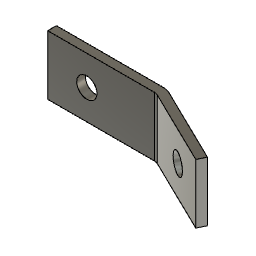
bracket154(2) (Autodesk Fusion 360 design; units mm, degrees)
Autodesk Fusion 360 part; units mm, degrees
sketch "Sketch1" plane through (0, 0, 0) normal (0, 0, 1) x (1, 0, 0)
  line L0 (0, 0) -> (0, -6)
  line L1 (0, -6) -> (75, -6)
  line L2 (75, -6) -> (128.0288, -31.8639)
  line L3 (128.0288, -31.8639) -> (130.6591, -26.4711)
  line L4 (0, 0) -> (76.3852, 0)
  line L5 (130.6591, -26.4711) -> (76.3852, 0)
  dimension "d9" = 6
  dimension "d10" = 75
  dimension "d11" = 59
  dimension "d12" = 154
  dimension "d13" = 6
  constraint coincident L0.start L4.start
  constraint vertical L0
  constraint perpendicular L0 L1
  constraint perpendicular L2 L3
  constraint perpendicular L0 L4
  constraint perpendicular L3 L5
  measures "d9" distance of L0.start L0.end
  measures "d10" distance of L0.end L1.end
  measures "d11" distance of L1.end L2.end
  measures "d12" angle of L1 L2
  measures "d13" distance of L2.end L3.end
extrude "Extrude1" add sketch "Sketch1" along normal blind 41
sketch "Sketch2" plane through (0, -6, 0) normal (0, -1, 0) x (1, 0, 0)
  line L0 (0, 0) -> (75, 0)
  line L1 (75, 0) -> (75, 41)
  line L2 (75, 41) -> (0, 41)
  line L3 (0, 41) -> (0, 0)
  circle A0 centre (27, 20.5) radius 7
  dimension "d16" = 14
  dimension "d17" = 27
  dimension "d18" = 20.5
  measures "d16" diameter of A0
  measures "d17" distance of L3 A0.centre
  measures "d18" distance of L0 A0.centre
extrude "Hole1" cut sketch "Sketch2" against normal blind 6 contours A0
sketch "Sketch3" plane through (12.0487, 24.7034, 0) normal (-0.438371, -0.898794, 0) x (0.898794, -0.438371, 0)
  line L0 (70.0398, 0) -> (129.0398, 0)
  line L1 (129.0398, 0) -> (129.0398, 41)
  line L2 (129.0398, 41) -> (70.0398, 41)
  line L3 (70.0398, 41) -> (70.0398, 0)
  circle A0 centre (102.0398, 20.5) radius 7
  dimension "d21" = 14
  dimension "d22" = 27
  dimension "d28" = 20.5
  measures "d21" diameter of A0
  measures "d22" distance of L1 A0.centre
  measures "d28" distance of L2 A0.centre
extrude "Hole2" cut sketch "Sketch3" against normal through all contours A0
fillet "Fillet1" radius 6 1 edges at (75, -6, 20.5)
fillet "Fillet1" radius 12 1 edges at (76.3852, 0, 20.5)
